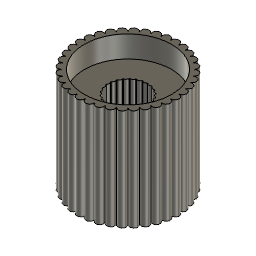
encoder_cap (Autodesk Fusion 360 design; units mm, degrees)
part number: 2026-01-18-21-15-22-192
Autodesk Fusion 360 part; units mm, degrees
sketch "Sketch1" plane through (0, 0, 0) normal (0, 0, 1) x (1, 0, 0)
  circle A0 centre (0, 0) radius 6.5
  dimension "d1" = 13
  constraint coincident A0.centre origin
  measures "d1" diameter of A0
extrude "Extrude1" add sketch "Sketch1" along normal blind 14
sketch "Sketch2" plane through (0, 0, 0) normal (0, 0, -1) x (1, 0, 0)
  circle A0 centre (0, 0) radius 6.5
  circle A1 centre (0, 0) radius 2.725
  dimension "d4" = 5.45
  constraint concentric A0 A1
  measures "d4" diameter of A1
extrude "Extrude2" cut sketch "Sketch2" against normal blind 12 contours A1
sketch "Sketch3" plane through (0, 0, 0) normal (0, 0, -1) x (1, 0, 0)
  circle A0 centre (0, 0) radius 2.725
  circle A1 centre (0, 0) radius 6.5
  circle A2 centre (0, 0) radius 2.925
  line L0 (-7.5, 0) -> (7.5, 0) construction
  circle A3 centre (-2.925, 0) radius 0.35
  circle A4 centre (-2.925, 0) radius 0.35
  circle A5 centre (-2.925, 0) radius 0.35
  circle A6 centre (-2.925, 0) radius 0.35
  circle A7 centre (-2.925, 0) radius 0.35
  circle A8 centre (-2.925, 0) radius 0.35
  circle A9 centre (-2.925, 0) radius 0.35
  circle A10 centre (-2.925, 0) radius 0.35
  circle A11 centre (-2.925, 0) radius 0.35
  circle A12 centre (-2.925, 0) radius 0.35
  circle A13 centre (-2.925, 0) radius 0.35
  circle A14 centre (-2.925, 0) radius 0.35
  circle A15 centre (-2.925, 0) radius 0.35
  circle A16 centre (-2.925, 0) radius 0.35
  circle A17 centre (-2.925, 0) radius 0.35
  circle A18 centre (-2.925, 0) radius 0.35
  circle A19 centre (-2.925, 0) radius 0.35
  circle A20 centre (-2.925, 0) radius 0.35
  circle A21 centre (-2.925, 0) radius 0.35
  circle A22 centre (-2.925, 0) radius 0.35
  circle A23 centre (-2.925, 0) radius 0.35
  circle A24 centre (-2.925, 0) radius 0.35
  circle A25 centre (-2.925, 0) radius 0.35
  circle A26 centre (-2.925, 0) radius 0.35
  circle A27 centre (-2.925, 0) radius 0.35
  circle A28 centre (-2.925, 0) radius 0.35
  circle A29 centre (-2.925, 0) radius 0.35
  circle A30 centre (-2.925, 0) radius 0.35
  circle A31 centre (-2.925, 0) radius 0.35
  circle A32 centre (-2.925, 0) radius 0.35
  circle A33 centre (-2.925, 0) radius 0.35
  circle A34 centre (-2.925, 0) radius 0.35
  circle A35 centre (-2.84, -0.7) radius 0.35
  circle A36 centre (-2.59, -1.3593) radius 0.35
  circle A37 centre (-2.1894, -1.9396) radius 0.35
  circle A38 centre (-1.6616, -2.4072) radius 0.35
  circle A39 centre (-1.0372, -2.7349) radius 0.35
  circle A40 centre (-0.3526, -2.9037) radius 0.35
  circle A41 centre (0.3526, -2.9037) radius 0.35
  circle A42 centre (1.0372, -2.7349) radius 0.35
  circle A43 centre (1.6616, -2.4072) radius 0.35
  circle A44 centre (2.1894, -1.9396) radius 0.35
  circle A45 centre (2.59, -1.3593) radius 0.35
  circle A46 centre (2.84, -0.7) radius 0.35
  circle A47 centre (2.925, 0) radius 0.35
  circle A48 centre (2.84, 0.7) radius 0.35
  circle A49 centre (2.59, 1.3593) radius 0.35
  circle A50 centre (2.1894, 1.9396) radius 0.35
  circle A51 centre (1.6616, 2.4072) radius 0.35
  circle A52 centre (1.0372, 2.7349) radius 0.35
  circle A53 centre (0.3526, 2.9037) radius 0.35
  circle A54 centre (-0.3526, 2.9037) radius 0.35
  circle A55 centre (-1.0372, 2.7349) radius 0.35
  circle A56 centre (-1.6616, 2.4072) radius 0.35
  circle A57 centre (-2.1894, 1.9396) radius 0.35
  circle A58 centre (-2.59, 1.3593) radius 0.35
  circle A59 centre (-2.84, 0.7) radius 0.35
  dimension "d7" = 0.2
  dimension "d8" = 0.7
  dimension "d10" = 360
  dimension "d12" = 360
  constraint horizontal L0
  constraint coincident L0 A3.centre
  constraint coincident A2 A3.centre
  measures "d8" diameter of A3
extrude "Extrude3" add sketch "Sketch3" against normal blind 12 contours A0 A47 | A0 A48 | A0 A46 | A0 A49 | A0 A45 | A0 A50 | A0 A44 | A0 A51 | A0 A43 | A0 A52 | A0 A42 | A0 A53 | A0 A41 | A0 A54 | A0 A40 | A0 A55 | A0 A39 | A0 A56 | A0 A38 | A0 A57 | A0 A37 | A0 A58 | A0 A36 | A0 A59 | A0 A35 | A0 A3 A4 A5 A6 A7 A8 A9 A10 A11 A12 A13 A14 A15 A16 A17 A18 A19 A20 A21 A22 A23 A24 A25 A26 A27 A28 A29 A30 A31 A32 A33 A34
sketch "Sketch4" plane through (0, 0, 14) normal (0, 0, 1) x (-1, 0, 0)
  circle A0 centre (0, 0) radius 6.5
  circle A1 centre (0, 0) radius 6
  dimension "d15" = 12
  constraint concentric A0 A1
  measures "d15" diameter of A1
extrude "Extrude4" cut sketch "Sketch4" against normal blind 2 contours A1
extrude "Extrude5" cut 1 faces at (3.3283, 3.5923, 12) along direction (0, 0, -1) blind 1
sketch "Sketch5" plane through (0, 0, 0) normal (0, 0, -1) x (1, 0, 0)
  arc A0 (-2.7109, -0.2769) -> (-2.6984, -0.3799) centre (0, 0) ccw
  arc A1 (-2.7109, -0.2769) -> (-2.7109, 0.2769) centre (-2.925, 0) ccw
  arc A2 (-2.6984, 0.3799) -> (-2.7109, 0.2769) centre (0, 0) ccw
  arc A3 (-2.6984, 0.3799) -> (-2.5659, 0.9176) centre (-2.84, 0.7) ccw
  arc A4 (-2.5291, 1.0147) -> (-2.5659, 0.9176) centre (0, 0) ccw
  arc A5 (-2.5291, 1.0147) -> (-2.2717, 1.505) centre (-2.59, 1.3593) ccw
  arc A6 (-2.2127, 1.5904) -> (-2.2717, 1.505) centre (0, 0) ccw
  arc A7 (-2.2127, 1.5904) -> (-1.8455, 2.0049) centre (-2.1894, 1.9396) ccw
  arc A8 (-1.7678, 2.0737) -> (-1.8455, 2.0049) centre (0, 0) ccw
  arc A9 (-1.7678, 2.0737) -> (-1.3121, 2.3883) centre (-1.6616, 2.4072) ccw
  arc A10 (-1.2202, 2.4366) -> (-1.3121, 2.3883) centre (0, 0) ccw
  arc A11 (-1.2202, 2.4366) -> (-0.7024, 2.6329) centre (-1.0372, 2.7349) ccw
  arc A12 (-0.6016, 2.6578) -> (-0.7024, 2.6329) centre (0, 0) ccw
  arc A13 (-0.6016, 2.6578) -> (-0.0519, 2.7245) centre (-0.3526, 2.9037) ccw
  arc A14 (0.0519, 2.7245) -> (-0.0519, 2.7245) centre (0, 0) ccw
  arc A15 (0.0519, 2.7245) -> (0.6016, 2.6578) centre (0.3526, 2.9037) ccw
  arc A16 (0.7024, 2.6329) -> (0.6016, 2.6578) centre (0, 0) ccw
  arc A17 (0.7024, 2.6329) -> (1.2202, 2.4366) centre (1.0372, 2.7349) ccw
  arc A18 (1.3121, 2.3883) -> (1.2202, 2.4366) centre (0, 0) ccw
  arc A19 (1.3121, 2.3883) -> (1.7678, 2.0737) centre (1.6616, 2.4072) ccw
  arc A20 (1.8455, 2.0049) -> (1.7678, 2.0737) centre (0, 0) ccw
  arc A21 (1.8455, 2.0049) -> (2.2127, 1.5904) centre (2.1894, 1.9396) ccw
  arc A22 (2.2717, 1.505) -> (2.2127, 1.5904) centre (0, 0) ccw
  arc A23 (2.2717, 1.505) -> (2.5291, 1.0147) centre (2.59, 1.3593) ccw
  arc A24 (2.5659, 0.9176) -> (2.5291, 1.0147) centre (0, 0) ccw
  arc A25 (2.5659, 0.9176) -> (2.6984, 0.3799) centre (2.84, 0.7) ccw
  arc A26 (2.7109, 0.2769) -> (2.6984, 0.3799) centre (0, 0) ccw
  arc A27 (2.7109, 0.2769) -> (2.7109, -0.2769) centre (2.925, 0) ccw
  arc A28 (2.6984, -0.3799) -> (2.7109, -0.2769) centre (0, 0) ccw
  arc A29 (2.6984, -0.3799) -> (2.5659, -0.9176) centre (2.84, -0.7) ccw
  arc A30 (2.5291, -1.0147) -> (2.5659, -0.9176) centre (0, 0) ccw
  arc A31 (2.5291, -1.0147) -> (2.2717, -1.505) centre (2.59, -1.3593) ccw
  arc A32 (2.2127, -1.5904) -> (2.2717, -1.505) centre (0, 0) ccw
  arc A33 (2.2127, -1.5904) -> (1.8455, -2.0049) centre (2.1894, -1.9396) ccw
  arc A34 (1.7678, -2.0737) -> (1.8455, -2.0049) centre (0, 0) ccw
  arc A35 (1.7678, -2.0737) -> (1.3121, -2.3883) centre (1.6616, -2.4072) ccw
  arc A36 (1.2202, -2.4366) -> (1.3121, -2.3883) centre (0, 0) ccw
  arc A37 (1.2202, -2.4366) -> (0.7024, -2.6329) centre (1.0372, -2.7349) ccw
  arc A38 (0.6016, -2.6578) -> (0.7024, -2.6329) centre (0, 0) ccw
  arc A39 (0.6016, -2.6578) -> (0.0519, -2.7245) centre (0.3526, -2.9037) ccw
  arc A40 (-0.0519, -2.7245) -> (0.0519, -2.7245) centre (0, 0) ccw
  arc A41 (-0.0519, -2.7245) -> (-0.6016, -2.6578) centre (-0.3526, -2.9037) ccw
  arc A42 (-0.7024, -2.6329) -> (-0.6016, -2.6578) centre (0, 0) ccw
  arc A43 (-0.7024, -2.6329) -> (-1.2202, -2.4366) centre (-1.0372, -2.7349) ccw
  arc A44 (-1.3121, -2.3883) -> (-1.2202, -2.4366) centre (0, 0) ccw
  arc A45 (-1.3121, -2.3883) -> (-1.7678, -2.0737) centre (-1.6616, -2.4072) ccw
  arc A46 (-1.8455, -2.0049) -> (-1.7678, -2.0737) centre (0, 0) ccw
  arc A47 (-1.8455, -2.0049) -> (-2.2127, -1.5904) centre (-2.1894, -1.9396) ccw
  arc A48 (-2.2717, -1.505) -> (-2.2127, -1.5904) centre (0, 0) ccw
  arc A49 (-2.2717, -1.505) -> (-2.5291, -1.0147) centre (-2.59, -1.3593) ccw
  arc A50 (-2.5659, -0.9176) -> (-2.5291, -1.0147) centre (0, 0) ccw
  arc A51 (-2.5659, -0.9176) -> (-2.6984, -0.3799) centre (-2.84, -0.7) ccw
  circle A52 centre (0, 0) radius 6.5
  circle A53 centre (0, -6.5) radius 0.55
  circle A54 centre (1.1287, -6.4013) radius 0.55
  circle A55 centre (2.2231, -6.108) radius 0.55
  circle A56 centre (3.25, -5.6292) radius 0.55
  circle A57 centre (4.1781, -4.9793) radius 0.55
  circle A58 centre (4.9793, -4.1781) radius 0.55
  circle A59 centre (5.6292, -3.25) radius 0.55
  circle A60 centre (6.108, -2.2231) radius 0.55
  circle A61 centre (6.4013, -1.1287) radius 0.55
  circle A62 centre (6.5, 0) radius 0.55
  circle A63 centre (6.4013, 1.1287) radius 0.55
  circle A64 centre (6.108, 2.2231) radius 0.55
  circle A65 centre (5.6292, 3.25) radius 0.55
  circle A66 centre (4.9793, 4.1781) radius 0.55
  circle A67 centre (4.1781, 4.9793) radius 0.55
  circle A68 centre (3.25, 5.6292) radius 0.55
  circle A69 centre (2.2231, 6.108) radius 0.55
  circle A70 centre (1.1287, 6.4013) radius 0.55
  circle A71 centre (0, 6.5) radius 0.55
  circle A72 centre (-1.1287, 6.4013) radius 0.55
  circle A73 centre (-2.2231, 6.108) radius 0.55
  circle A74 centre (-3.25, 5.6292) radius 0.55
  circle A75 centre (-4.1781, 4.9793) radius 0.55
  circle A76 centre (-4.9793, 4.1781) radius 0.55
  circle A77 centre (-5.6292, 3.25) radius 0.55
  circle A78 centre (-6.108, 2.2231) radius 0.55
  circle A79 centre (-6.4013, 1.1287) radius 0.55
  circle A80 centre (-6.5, 0) radius 0.55
  circle A81 centre (-6.4013, -1.1287) radius 0.55
  circle A82 centre (-6.108, -2.2231) radius 0.55
  circle A83 centre (-5.6292, -3.25) radius 0.55
  circle A84 centre (-4.9793, -4.1781) radius 0.55
  circle A85 centre (-4.1781, -4.9793) radius 0.55
  circle A86 centre (-3.25, -5.6292) radius 0.55
  circle A87 centre (-2.2231, -6.108) radius 0.55
  circle A88 centre (-1.1287, -6.4013) radius 0.55
  dimension "d22" = 1.1
  dimension "d24" = 360
  constraint coincident A52 A53.centre
  measures "d22" diameter of A53
extrude "Extrude6" add sketch "Sketch5" against normal blind 14 contours A52 A62 | A52 A63 | A52 A61 | A52 A64 | A52 A60 | A52 A65 | A52 A59 | A52 A66 | A52 A58 | A52 A67 | A52 A57 | A52 A68 | A52 A56 | A52 A69 | A52 A55 | A52 A70 | A52 A54 | A52 A71 | A52 A53 | A52 A72 | A52 A88 | A52 A73 | A52 A87 | A52 A74 | A52 A86 | A52 A75 | A52 A85 | A52 A76 | A52 A84 | A52 A77 | A52 A83 | A52 A78 | A52 A82 | A52 A79 | A52 A81 | A52 A80 picked at (6.6746, -0.1141) picked at (6.5809, 1.1556) picked at (6.5809, -1.1556) picked at (6.2826, 2.2733) picked at (6.2826, -2.2733) picked at (5.782, 3.348) picked at (5.782, -3.348) picked at (5.1155, 4.2982) picked at (5.1155, -4.2982) picked at (4.2942, 5.119) picked at (4.2942, -5.119) picked at (3.3428, 5.7853) picked at (3.3428, -5.7853) picked at (2.2901, 6.2768) picked at (2.2901, -6.2768) picked at (1.1536, 6.5811) picked at (1.1536, -6.5811) picked at (-0.0039, 6.6816) picked at (-0.0039, -6.6816) picked at (-1.1602, 6.5801) picked at (-1.1602, -6.5801) picked at (-2.2852, 6.2787) picked at (-2.2852, -6.2787) picked at (-3.3408, 5.7864) picked at (-3.3408, -5.7864) picked at (-4.2949, 5.1184) picked at (-4.2949, -5.1184) picked at (-5.1184, 4.2949) picked at (-5.1184, -4.2949) picked at (-5.7864, 3.3408) picked at (-5.7864, -3.3408) picked at (-6.2787, 2.2852) picked at (-6.2787, -2.2852) picked at (-6.5801, 1.1602) picked at (-6.5801, -1.1602) picked at (-6.6816, 0)
